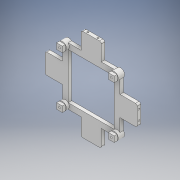
# Autodesk Inventor part: solar roof
Saved by Autodesk Inventor 2017 (Build 210142000, 142)
## iProperties
Created: 2019-02-02
Part Number: solar roof
Material: ABS Plastic
Document SubType Name: Modeling
Designer: simulator
Density: 1.06 g/cm^3
Appearance: Smooth - White
Mass: 52.751 g
Surface Area: 242.7 cm^2
Volume: 49.7651 cm^3
Author: simulator
Autodesk Inventor part; units mm, degrees
ref_plane "YZ Plane" through (0, 0, 0) normal (1, 0, 0) x (0, 1, 0)
ref_plane "XZ Plane" through (0, 0, 0) normal (0, 1, 0) x (-1, 0, 0)
ref_plane "XY Plane" through (0, 0, 0) normal (0, 0, 1) x (1, 0, 0)
sketch "Sketch1" plane through (0, 0, 0) normal (0, 1, 0) x (-1, 0, 0)
  line L0 (-36.5, 50) -> (-36.5, 45)
  circle A0 centre (45, 45) radius 1.5
  circle A1 centre (-45, -45) radius 1.5
  circle A2 centre (45, -45) radius 1.5
  circle A3 centre (-45, 45) radius 1.5
  line L1 (-50, 50) -> (50, 50)
  line L2 (-50, -50) -> (-50, 50)
  line L3 (50, -50) -> (-50, -50)
  line L4 (50, 50) -> (50, -50)
  line L5 (40, 45) -> (-40, 45)
  line L6 (40, 40) -> (40, 45)
  line L7 (45, 40) -> (40, 40)
  line L8 (45, -40) -> (45, 40)
  line L9 (40, -40) -> (45, -40)
  line L10 (40, -45) -> (40, -40)
  line L11 (-40, -45) -> (40, -45)
  line L12 (-40, -40) -> (-40, -45)
  line L13 (-45, -40) -> (-40, -40)
  line L14 (-45, 40) -> (-45, -40)
  line L15 (-40, 40) -> (-45, 40)
  line L16 (-40, 45) -> (-40, 40)
  line L17 (50, 50) -> (40, 50)
  line L18 (40, 50) -> (40, -50)
  line L19 (40, -50) -> (50, -50)
  line L20 (50, -50) -> (50, 50)
  line L21 (-82.5, 82.5) -> (-82.5, -82.5)
  line L22 (80, 17.5) -> (40, 17.5)
  line L23 (40, 17.5) -> (40, -17.5)
  line L24 (40, -17.5) -> (80, -17.5)
  line L25 (80, -17.5) -> (80, 17.5)
  point P0 (0, 0)
  point P1 (0, 0)
  point P2 (0, 0)
  point P3 (40, 0)
  point P4 (80, 0)
  dimension "d3" = 35
  dimension "d19" = 40
  constraints: 52 end point, 4 centre point, 4 parallel, 3 midpoint, 2 horizontal, 2 perpendicular, 1 coincident, 1 point on line
  measures "d3" distance between parallel lines of L22 L24
  measures "d19" distance of L23.end L24.end
extrude "Extrusion1" add sketch "Sketch1" along normal blind 6 contours L1 L4 L22 L8 L7 L6 L18 | L7 L8 L22 L18 | L18 L10 L9 L8 L24 L4 L3 | L22 L25 L24 L4 | L4 L24 L8 L22 | L22 L8 L24 L18 | L24 L8 L9 L18
pattern_circular "Circular Pattern1" count 4 over 360 about axis through (0, -10, 0) along (0, 1, 0) of "Extrusion1"
sketch "Sketch2" plane through (80, 0, 17.5) normal (1, 0, 0) x (0, 0, -1)
  line L0 (0, 0) -> (35, 0) projected
  line L1 (35, 0) -> (35, 6) projected
  line L2 (0, 6) -> (35, 6) projected
  line L3 (0, 0) -> (0, 6) projected
  line L4 (0, 6) -> (0, 0) projected
  line L5 (0, 3) -> (35, 3)
  line L6 (17.5, 3) -> (35, 3)
  line L7 (17.5, 3) -> (0, 3)
  point P0 (17.5, 0)
  point P1 (8.75, 3)
  point P2 (26.25, 3)
  constraints: 6 end point, 5 midpoint, 2 collinear
hole "Hole1" at (80, 3, 8.75) at (80, 3, -8.75) direction (-1, 0, 0) diameter 3 depth 10 tip angle 118
pattern_circular "Circular Pattern2" count 4 over 360 about axis through (0, -10, 0) along (0, 1, 0) of "Hole1"
sketch "Sketch3" plane through (0, 0, 0) normal (0, -1, 0) x (1, 0, 0)
  line L0 (-50, -50) -> (-40, -50)
  line L1 (-40, -50) -> (-40, -40)
  line L2 (-40, -40) -> (-50, -40)
  line L3 (-50, -40) -> (-50, -50)
  line L4 (50, -50) -> (40, -50)
  line L5 (40, -50) -> (40, -40)
  line L6 (40, -40) -> (50, -40)
  line L7 (50, -40) -> (50, -50)
  line L8 (50, 50) -> (40, 50)
  line L9 (40, 50) -> (40, 40)
  line L10 (40, 40) -> (50, 40)
  line L11 (50, 40) -> (50, 50)
  line L12 (-50, 50) -> (-17.5, 50) projected
  line L13 (-50, 50) -> (-40, 50)
  line L14 (-40, 50) -> (-40, 40)
  line L15 (-40, 40) -> (-50, 40)
  line L16 (-50, 40) -> (-50, 50)
  circle A0 centre (-45, 45) radius 1.5 projected
  circle A1 centre (45, 45) radius 1.5 projected
  circle A2 centre (-45, -45) radius 1.5 projected
  circle A3 centre (45, -45) radius 1.5 projected
  circle A4 centre (45, 45) radius 7.0711
  line L17 (-40, 40) -> (-40, -40) projected
  circle A5 centre (-45, 45) radius 7.0711
  circle A6 centre (-45, -45) radius 7.0711
  line L18 (50, -50) -> (17.5, -50) projected
  circle A7 centre (45, -45) radius 7.0711
  point P0 (0, 0)
  dimension "d20" = 10
  dimension "d21" = 10
  dimension "d22" = 10
  dimension "d23" = 10
  dimension "d24" = 10
  dimension "d25" = 10
  dimension "d26" = 10
  dimension "d27" = 10
  constraints: 32 end point, 8 parallel, 4 coincident, 4 horizontal, 4 perpendicular, 12 other
  measures "d20" distance of L2.end L1.end
  measures "d21" distance of L1.end L0.end
  measures "d22" distance of L5.end L6.end
  measures "d23" distance of L4.end L5.end
  measures "d24" distance of L10.end L9.end
  measures "d25" distance of L9.end L8.end
  measures "d26" distance of L14.end L15.end
  measures "d27" distance of L13.end L14.end
extrude "Extrusion2" add sketch "Sketch3" along normal blind 5 and the other way blind 6
fillet "Fillet4" radius 3 8 edges at (-17.5, 3, 80) (-80, 3, 17.5) (-80, 3, -17.5) (-17.5, 3, -80) (17.5, 3, -80) (80, 3, -17.5) (80, 3, 17.5) (17.5, 3, 80)
extrude "Extrusion3" add sketch "Sketch3" along normal blind 10 contours L3 L2 L1 L0 | L15 L16 L12 L14 | L4 L5 L6 L7 | L11 L10 L9 L8
body "Solid1"
